Autodesk Fusion 360 part; units mm, degrees
note: some values were not read from the file. Set by a fixed rule: which sketch regions a step uses.
(part 37 of 59)
  spline S18 degree 5 poles (-22.1904, -6.2406) (-22.1905, -6.2407) (-22.1907, -6.2408) (-22.1909, -6.241) (-22.1913, -6.2414) (-22.1919, -6.2419) (-22.1925, -6.2424) (-22.1933, -6.2431) (-22.1941, -6.2438) (-22.195, -6.2446) (-22.196, -6.2455) (-22.197, -6.2464) (-22.1982, -6.2474) (-22.1994, -6.2485) (-22.2007, -6.2497) (-22.202, -6.2509) (-22.2035, -6.2522) (-22.205, -6.2536) (-22.2066, -6.255) (-22.2082, -6.2565) (-22.2099, -6.2581) (-22.2117, -6.2597) (-22.2136, -6.2615) (-22.2155, -6.2632) (-22.2175, -6.2651) (-22.2195, -6.267) (-22.2216, -6.269) (-22.2238, -6.271) (-22.226, -6.2732) (-22.2283, -6.2753) (-22.2307, -6.2776) (-22.2331, -6.2799) (-22.2355, -6.2823) (-22.238, -6.2847) (-22.2406, -6.2872) (-22.2433, -6.2897) (-22.2459, -6.2924) (-22.2487, -6.2951) (-22.2515, -6.2978) (-22.2543, -6.3006) (-22.2572, -6.3035) (-22.2602, -6.3064) (-22.2632, -6.3094) (-22.2662, -6.3124) (-22.2693, -6.3156) (-22.2725, -6.3187) (-22.2757, -6.322) (-22.2789, -6.3252) (-22.2822, -6.3286) (-22.2855, -6.332) (-22.2889, -6.3355) (-22.2923, -6.339) (-22.2958, -6.3426) (-22.2993, -6.3462) (-22.3029, -6.3499) (-22.3065, -6.3536) (-22.3101, -6.3574) (-22.3138, -6.3613) (-22.3175, -6.3652) (-22.3212, -6.3692) (-22.325, -6.3732) (-22.3289, -6.3773) (-22.3328, -6.3814) (-22.3367, -6.3856) (-22.3406, -6.3899) (-22.3446, -6.3942) (-22.3486, -6.3986) (-22.3527, -6.403) (-22.3568, -6.4074) (-22.3609, -6.4119) (-22.3651, -6.4165) (-22.3693, -6.4211) (-22.3736, -6.4258) (-22.3778, -6.4306) (-22.3821, -6.4353) (-22.3865, -6.4402) (-22.3909, -6.4451) (-22.3953, -6.45) (-22.3997, -6.455) (-22.4042, -6.46) (-22.4087, -6.4651) (-22.4132, -6.4703) (-22.4177, -6.4755) (-22.4223, -6.4807) (-22.427, -6.486) (-22.4316, -6.4914) (-22.4363, -6.4968) (-22.441, -6.5022) (-22.4457, -6.5077) (-22.4505, -6.5133) (-22.4553, -6.5189) (-22.4601, -6.5246) (-22.4649, -6.5303) (-22.4698, -6.536) (-22.4747, -6.5418) (-22.4796, -6.5477) (-22.4846, -6.5536) (-22.4895, -6.5595) (-22.4945, -6.5655) (-22.4996, -6.5715) (-22.5046, -6.5776) (-22.5097, -6.5838) (-22.5148, -6.59) (-22.5199, -6.5962) (-22.525, -6.6025) (-22.5302, -6.6088) (-22.5354, -6.6152) (-22.5406, -6.6216) (-22.5458, -6.6281) (-22.5511, -6.6346) (-22.5564, -6.6412) (-22.5617, -6.6478) (-22.567, -6.6544) (-22.5723, -6.6611) (-22.5777, -6.6679) (-22.583, -6.6747) (-22.5884, -6.6815) (-22.5939, -6.6884) (-22.5993, -6.6954) (-22.6048, -6.7024) (-22.6102, -6.7094) (-22.6157, -6.7165) (-22.6212, -6.7236) (-22.6268, -6.7307) (-22.6323, -6.7379) (-22.6379, -6.7452) (-22.6435, -6.7525) (-22.6491, -6.7598) (-22.6547, -6.7672) (-22.6603, -6.7747) (-22.666, -6.7821) (-22.6716, -6.7897) (-22.6773, -6.7972) (-22.683, -6.8048) (-22.6887, -6.8125) (-22.6945, -6.8202) (-22.7002, -6.8279) (-22.706, -6.8357) (-22.7118, -6.8436) (-22.7175, -6.8514) (-22.7233, -6.8593) (-22.7292, -6.8673) (-22.735, -6.8753) (-22.7408, -6.8834) (-22.7467, -6.8914) (-22.7526, -6.8996) (-22.7585, -6.9078) (-22.7644, -6.916) (-22.7703, -6.9242) (-22.7762, -6.9325) (-22.7822, -6.9409) (-22.7881, -6.9493) (-22.7941, -6.9577) (-22.8, -6.9662) (-22.806, -6.9747) (-22.812, -6.9832) (-22.818, -6.9918) (-22.8241, -7.0005) (-22.8301, -7.0091) (-22.8361, -7.0179) (-22.8422, -7.0266) (-22.8483, -7.0354) (-22.8543, -7.0443) (-22.8604, -7.0532) (-22.8665, -7.0621) (-22.8726, -7.0711) (-22.8787, -7.0801) (-22.8849, -7.0891) (-22.891, -7.0982) (-22.8971, -7.1073) (-22.9033, -7.1165) (-22.9095, -7.1257) (-22.9156, -7.135) (-22.9218, -7.1443) (-22.928, -7.1536) (-22.9342, -7.163) (-22.9404, -7.1724) (-22.9466, -7.1818) (-22.9528, -7.1913) (-22.9591, -7.2009) (-22.9653, -7.2104) (-22.9715, -7.22) (-22.9778, -7.2297) (-22.984, -7.2394) (-22.9903, -7.2491) (-22.9966, -7.2589) (-23.0029, -7.2687) (-23.0091, -7.2785) (-23.0154, -7.2884) (-23.0217, -7.2984) (-23.028, -7.3083) (-23.0343, -7.3183) (-23.0406, -7.3284) (-23.047, -7.3384) (-23.0533, -7.3486) (-23.0596, -7.3587) (-23.066, -7.3689) (-23.0723, -7.3791) (-23.0786, -7.3894) (-23.085, -7.3997) (-23.0914, -7.4101) (-23.0977, -7.4205) (-23.1041, -7.4309) (-23.1104, -7.4413) (-23.1168, -7.4518) (-23.1232, -7.4624) (-23.1296, -7.473) (-23.136, -7.4836) (-23.1423, -7.4942) (-23.1487, -7.5049) (-23.1551, -7.5156) (-23.1615, -7.5264) (-23.1679, -7.5372) (-23.1743, -7.548) (-23.1807, -7.5589) (-23.1872, -7.5698) (-23.1936, -7.5808) (-23.2, -7.5917) (-23.2064, -7.6028) (-23.2128, -7.6138) (-23.2193, -7.6249) (-23.2257, -7.636) (-23.2321, -7.6472) (-23.2385, -7.6584) (-23.245, -7.6697) (-23.2514, -7.6809) (-23.2578, -7.6922) (-23.2643, -7.7036) (-23.2707, -7.715) (-23.2771, -7.7264) (-23.2836, -7.7379) (-23.29, -7.7493) (-23.2965, -7.7609) (-23.3029, -7.7724) (-23.3094, -7.784) (-23.3158, -7.7957) (-23.3222, -7.8073) (-23.3287, -7.819) (-23.3351, -7.8308) (-23.3416, -7.8426) (-23.348, -7.8544) (-23.3532, -7.8639) (-23.3571, -7.871) (-23.3596, -7.8757) (-23.3609, -7.8781) knots 0 0 0 0 0 0 0.00416667 0.00833333 0.0125 0.01666667 0.02083333 0.025 0.02916667 0.03333333 0.0375 0.04166667 0.04583333 0.05 0.05416667 0.05833333 0.0625 0.06666667 0.07083333 0.075 0.07916667 0.08333333 0.0875 0.09166667 0.09583333 0.1 0.10416667 0.10833333 0.1125 0.11666667 0.12083333 0.125 0.12916667 0.13333333 0.1375 0.14166667 0.14583333 0.15 0.15416667 0.15833333 0.1625 0.16666667 0.17083333 0.175 0.17916667 0.18333333 0.1875 0.19166667 0.19583333 0.2 0.20416667 0.20833333 0.2125 0.21666667 0.22083333 0.225 0.22916667 0.23333333 0.2375 0.24166667 0.24583333 0.25 0.25416667 0.25833333 0.2625 0.26666667 0.27083333 0.275 0.27916667 0.28333333 0.2875 0.29166667 0.29583333 0.3 0.30416667 0.30833333 0.3125 0.31666667 0.32083333 0.325 0.32916667 0.33333333 0.3375 0.34166667 0.34583333 0.35 0.35416667 0.35833333 0.3625 0.36666667 0.37083333 0.375 0.37916667 0.38333333 0.3875 0.39166667 0.39583333 0.4 0.40416667 0.40833333 0.4125 0.41666667 0.42083333 0.425 0.42916667 0.43333333 0.4375 0.44166667 0.44583333 0.45 0.45416667 0.45833333 0.4625 0.46666667 0.47083333 0.475 0.47916667 0.48333333 0.4875 0.49166667 0.49583333 0.5 0.50416667 0.50833333 0.5125 0.51666667 0.52083333 0.525 0.52916667 0.53333333 0.5375 0.54166667 0.54583333 0.55 0.55416667 0.55833333 0.5625 0.56666667 0.57083333 0.575 0.57916667 0.58333333 0.5875 0.59166667 0.59583333 0.6 0.60416667 0.60833333 0.6125 0.61666667 0.62083333 0.625 0.62916667 0.63333333 0.6375 0.64166667 0.64583333 0.65 0.65416667 0.65833333 0.6625 0.66666667 0.67083333 0.675 0.67916667 0.68333333 0.6875 0.69166667 0.69583333 0.7 0.70416667 0.70833333 0.7125 0.71666667 0.72083333 0.725 0.72916667 0.73333333 0.7375 0.74166667 0.74583333 0.75 0.75416667 0.75833333 0.7625 0.76666667 0.77083333 0.775 0.77916667 0.78333333 0.7875 0.79166667 0.79583333 0.8 0.80416667 0.80833333 0.8125 0.81666667 0.82083333 0.825 0.82916667 0.83333333 0.8375 0.84166667 0.84583333 0.85 0.85416667 0.85833333 0.8625 0.86666667 0.87083333 0.875 0.87916667 0.88333333 0.8875 0.89166667 0.89583333 0.9 0.90416667 0.90833333 0.9125 0.91666667 0.92083333 0.925 0.92916667 0.93333333 0.9375 0.94166667 0.94583333 0.95 0.95416667 0.95833333 0.9625 0.96666667 0.97083333 0.975 0.97916667 0.98333333 0.9875 0.99166667 0.99583333 1 1 1 1 1 1
  arc A19 (-23.3609, -7.8781) -> (-22.7084, -8.6029) centre (0, 12.5) ccw
  spline S19 degree 5 poles (-22.7084, -8.6029) (-22.7059, -8.6018) (-22.7009, -8.5998) (-22.6934, -8.5967) (-22.6834, -8.5925) (-22.671, -8.5873) (-22.6586, -8.5822) (-22.6462, -8.577) (-22.6339, -8.5718) (-22.6217, -8.5666) (-22.6094, -8.5614) (-22.5972, -8.5562) (-22.585, -8.551) (-22.5729, -8.5458) (-22.5608, -8.5406) (-22.5487, -8.5354) (-22.5367, -8.5302) (-22.5247, -8.525) (-22.5127, -8.5198) (-22.5008, -8.5145) (-22.4889, -8.5093) (-22.4771, -8.5041) (-22.4653, -8.4989) (-22.4535, -8.4937) (-22.4417, -8.4884) (-22.43, -8.4832) (-22.4184, -8.478) (-22.4067, -8.4727) (-22.3951, -8.4675) (-22.3836, -8.4623) (-22.3721, -8.457) (-22.3606, -8.4518) (-22.3491, -8.4466) (-22.3377, -8.4413) (-22.3264, -8.4361) (-22.315, -8.4308) (-22.3037, -8.4256) (-22.2925, -8.4204) (-22.2812, -8.4151) (-22.2701, -8.4099) (-22.2589, -8.4046) (-22.2478, -8.3994) (-22.2367, -8.3942) (-22.2257, -8.3889) (-22.2147, -8.3837) (-22.2038, -8.3784) (-22.1928, -8.3732) (-22.182, -8.368) (-22.1711, -8.3627) (-22.1603, -8.3575) (-22.1496, -8.3523) (-22.1388, -8.347) (-22.1281, -8.3418) (-22.1175, -8.3366) (-22.1069, -8.3313) (-22.0963, -8.3261) (-22.0858, -8.3209) (-22.0753, -8.3157) (-22.0649, -8.3105) (-22.0544, -8.3052) (-22.0441, -8.3) (-22.0337, -8.2948) (-22.0235, -8.2896) (-22.0132, -8.2844) (-22.003, -8.2792) (-21.9928, -8.274) (-21.9827, -8.2688) (-21.9726, -8.2636) (-21.9625, -8.2584) (-21.9525, -8.2532) (-21.9426, -8.248) (-21.9326, -8.2429) (-21.9228, -8.2377) (-21.9129, -8.2325) (-21.9031, -8.2274) (-21.8933, -8.2222) (-21.8836, -8.217) (-21.8739, -8.2119) (-21.8643, -8.2067) (-21.8547, -8.2016) (-21.8451, -8.1965) (-21.8356, -8.1913) (-21.8261, -8.1862) (-21.8167, -8.1811) (-21.8073, -8.176) (-21.798, -8.1709) (-21.7887, -8.1658) (-21.7794, -8.1607) (-21.7702, -8.1556) (-21.761, -8.1505) (-21.7519, -8.1454) (-21.7428, -8.1404) (-21.7337, -8.1353) (-21.7247, -8.1303) (-21.7158, -8.1252) (-21.7068, -8.1202) (-21.698, -8.1152) (-21.6891, -8.1101) (-21.6803, -8.1051) (-21.6716, -8.1001) (-21.6629, -8.0951) (-21.6542, -8.0902) (-21.6456, -8.0852) (-21.6371, -8.0802) (-21.6285, -8.0753) (-21.6201, -8.0703) (-21.6116, -8.0654) (-21.6032, -8.0605) (-21.5949, -8.0555) (-21.5866, -8.0506) (-21.5783, -8.0457) (-21.5701, -8.0409) (-21.5619, -8.036) (-21.5538, -8.0311) (-21.5458, -8.0263) (-21.5377, -8.0214) (-21.5297, -8.0166) (-21.5218, -8.0118) (-21.5139, -8.007) (-21.5061, -8.0022) (-21.4983, -7.9974) (-21.4905, -7.9927) (-21.4828, -7.9879) (-21.4752, -7.9832) (-21.4676, -7.9784) (-21.46, -7.9737) (-21.4525, -7.969) (-21.445, -7.9644) (-21.4376, -7.9597) (-21.4302, -7.955) (-21.4229, -7.9504) (-21.4156, -7.9458) (-21.4084, -7.9412) (-21.4012, -7.9366) (-21.3941, -7.932) (-21.387, -7.9274) (-21.38, -7.9229) (-21.373, -7.9184) (-21.3661, -7.9139) (-21.3592, -7.9094) (-21.3523, -7.9049) (-21.3455, -7.9004) (-21.3388, -7.896) (-21.3321, -7.8916) (-21.3255, -7.8872) (-21.3189, -7.8828) (-21.3124, -7.8784) (-21.3059, -7.8741) (-21.2995, -7.8698) (-21.2931, -7.8655) (-21.2867, -7.8612) (-21.2805, -7.8569) (-21.2742, -7.8527) (-21.2681, -7.8484) (-21.2619, -7.8442) (-21.2559, -7.8401) (-21.2498, -7.8359) (-21.2439, -7.8318) (-21.238, -7.8277) (-21.2321, -7.8236) (-21.2263, -7.8195) (-21.2205, -7.8155) (-21.2148, -7.8115) (-21.2092, -7.8075) (-21.2036, -7.8035) (-21.1981, -7.7996) (-21.1926, -7.7956) (-21.1871, -7.7918) (-21.1818, -7.7879) (-21.1764, -7.7841) (-21.1712, -7.7802) (-21.166, -7.7765) (-21.1608, -7.7727) (-21.1557, -7.769) (-21.1507, -7.7653) (-21.1457, -7.7616) (-21.1408, -7.758) (-21.1359, -7.7544) (-21.1311, -7.7508) (-21.1263, -7.7472) (-21.1216, -7.7437) (-21.117, -7.7402) (-21.1124, -7.7368) (-21.1079, -7.7333) (-21.1034, -7.73) (-21.099, -7.7266) (-21.0947, -7.7233) (-21.0904, -7.72) (-21.0862, -7.7167) (-21.082, -7.7135) (-21.0779, -7.7103) (-21.0739, -7.7072) (-21.0699, -7.7041) (-21.066, -7.701) (-21.0621, -7.698) (-21.0583, -7.695) (-21.0546, -7.692) (-21.0509, -7.6891) (-21.0473, -7.6862) (-21.0437, -7.6834) (-21.0403, -7.6806) (-21.0368, -7.6778) (-21.0335, -7.6751) (-21.0302, -7.6724) (-21.027, -7.6698) (-21.0238, -7.6672) (-21.0207, -7.6647) (-21.0177, -7.6622) (-21.0148, -7.6597) (-21.0119, -7.6573) (-21.009, -7.655) (-21.0063, -7.6527) (-21.0036, -7.6504) (-21.001, -7.6482) (-20.9984, -7.6461) (-20.996, -7.644) (-20.9936, -7.6419) (-20.9912, -7.6399) (-20.989, -7.638) (-20.9868, -7.6361) (-20.9847, -7.6343) (-20.9826, -7.6325) (-20.9806, -7.6308) (-20.9787, -7.6291) (-20.9769, -7.6275) (-20.9752, -7.626) (-20.9735, -7.6245) (-20.9719, -7.623) (-20.9704, -7.6217) (-20.9689, -7.6204) (-20.9675, -7.6192) (-20.9663, -7.618) (-20.9651, -7.6169) (-20.9639, -7.6159) (-20.9629, -7.6149) (-20.9619, -7.614) (-20.961, -7.6132) (-20.9602, -7.6125) (-20.9595, -7.6118) (-20.9589, -7.6112) (-20.9583, -7.6107) (-20.958, -7.6104) (-20.9577, -7.6102) (-20.9576, -7.61) (-20.9575, -7.61) knots -1 -1 -1 -1 -1 -1 -0.99583333 -0.99166667 -0.9875 -0.98333333 -0.97916667 -0.975 -0.97083333 -0.96666667 -0.9625 -0.95833333 -0.95416667 -0.95 -0.94583333 -0.94166667 -0.9375 -0.93333333 -0.92916667 -0.925 -0.92083333 -0.91666667 -0.9125 -0.90833333 -0.90416667 -0.9 -0.89583333 -0.89166667 -0.8875 -0.88333333 -0.87916667 -0.875 -0.87083333 -0.86666667 -0.8625 -0.85833333 -0.85416667 -0.85 -0.84583333 -0.84166667 -0.8375 -0.83333333 -0.82916667 -0.825 -0.82083333 -0.81666667 -0.8125 -0.80833333 -0.80416667 -0.8 -0.79583333 -0.79166667 -0.7875 -0.78333333 -0.77916667 -0.775 -0.77083333 -0.76666667 -0.7625 -0.75833333 -0.75416667 -0.75 -0.74583333 -0.74166667 -0.7375 -0.73333333 -0.72916667 -0.725 -0.72083333 -0.71666667 -0.7125 -0.70833333 -0.70416667 -0.7 -0.69583333 -0.69166667 -0.6875 -0.68333333 -0.67916667 -0.675 -0.67083333 -0.66666667 -0.6625 -0.65833333 -0.65416667 -0.65 -0.64583333 -0.64166667 -0.6375 -0.63333333 -0.62916667 -0.625 -0.62083333 -0.61666667 -0.6125 -0.60833333 -0.60416667 -0.6 -0.59583333 -0.59166667 -0.5875 -0.58333333 -0.57916667 -0.575 -0.57083333 -0.56666667 -0.5625 -0.55833333 -0.55416667 -0.55 -0.54583333 -0.54166667 -0.5375 -0.53333333 -0.52916667 -0.525 -0.52083333 -0.51666667 -0.5125 -0.50833333 -0.50416667 -0.5 -0.49583333 -0.49166667 -0.4875 -0.48333333 -0.47916667 -0.475 -0.47083333 -0.46666667 -0.4625 -0.45833333 -0.45416667 -0.45 -0.44583333 -0.44166667 -0.4375 -0.43333333 -0.42916667 -0.425 -0.42083333 -0.41666667 -0.4125 -0.40833333 -0.40416667 -0.4 -0.39583333 -0.39166667 -0.3875 -0.38333333 -0.37916667 -0.375 -0.37083333 -0.36666667 -0.3625 -0.35833333 -0.35416667 -0.35 -0.34583333 -0.34166667 -0.3375 -0.33333333 -0.32916667 -0.325 -0.32083333 -0.31666667 -0.3125 -0.30833333 -0.30416667 -0.3 -0.29583333 -0.29166667 -0.2875 -0.28333333 -0.27916667 -0.275 -0.27083333 -0.26666667 -0.2625 -0.25833333 -0.25416667 -0.25 -0.24583333 -0.24166667 -0.2375 -0.23333333 -0.22916667 -0.225 -0.22083333 -0.21666667 -0.2125 -0.20833333 -0.20416667 -0.2 -0.19583333 -0.19166667 -0.1875 -0.18333333 -0.17916667 -0.175 -0.17083333 -0.16666667 -0.1625 -0.15833333 -0.15416667 -0.15 -0.14583333 -0.14166667 -0.1375 -0.13333333 -0.12916667 -0.125 -0.12083333 -0.11666667 -0.1125 -0.10833333 -0.10416667 -0.1 -0.09583333 -0.09166667 -0.0875 -0.08333333 -0.07916667 -0.075 -0.07083333 -0.06666667 -0.0625 -0.05833333 -0.05416667 -0.05 -0.04583333 -0.04166667 -0.0375 -0.03333333 -0.02916667 -0.025 -0.02083333 -0.01666667 -0.0125 -0.00833333 -0.00416667 0 0 0 0 0 0
  line L47 (-20.9575, -7.61) -> (-20.9569, -7.6094)
  line L48 (-20.9569, -7.6094) -> (-20.7445, -7.4055)
  arc A20 (-20.7445, -7.4055) -> (-19.9055, -8.2445) centre (0, 12.5) ccw
  line L49 (-19.9055, -8.2445) -> (-20.1094, -8.4569)
  line L50 (-20.1094, -8.4569) -> (-20.11, -8.4575)
  spline S20 degree 5 poles (-20.11, -8.4575) (-20.11, -8.4576) (-20.1102, -8.4577) (-20.1104, -8.458) (-20.1107, -8.4583) (-20.1112, -8.4589) (-20.1118, -8.4595) (-20.1125, -8.4602) (-20.1132, -8.461) (-20.114, -8.4619) (-20.1149, -8.4629) (-20.1159, -8.4639) (-20.1169, -8.4651) (-20.118, -8.4663) (-20.1192, -8.4675) (-20.1204, -8.4689) (-20.1217, -8.4704) (-20.123, -8.4719) (-20.1245, -8.4735) (-20.126, -8.4752) (-20.1275, -8.4769) (-20.1291, -8.4787) (-20.1308, -8.4806) (-20.1325, -8.4826) (-20.1343, -8.4847) (-20.1361, -8.4868) (-20.138, -8.489) (-20.1399, -8.4912) (-20.1419, -8.4936) (-20.144, -8.496) (-20.1461, -8.4984) (-20.1482, -8.501) (-20.1504, -8.5036) (-20.1527, -8.5063) (-20.155, -8.509) (-20.1573, -8.5119) (-20.1597, -8.5148) (-20.1622, -8.5177) (-20.1647, -8.5207) (-20.1672, -8.5238) (-20.1698, -8.527) (-20.1724, -8.5302) (-20.1751, -8.5335) (-20.1778, -8.5368) (-20.1806, -8.5403) (-20.1834, -8.5437) (-20.1862, -8.5473) (-20.1891, -8.5509) (-20.192, -8.5546) (-20.195, -8.5583) (-20.198, -8.5621) (-20.201, -8.566) (-20.2041, -8.5699) (-20.2072, -8.5739) (-20.2103, -8.5779) (-20.2135, -8.582) (-20.2167, -8.5862) (-20.22, -8.5904) (-20.2233, -8.5947) (-20.2266, -8.599) (-20.23, -8.6034) (-20.2333, -8.6079) (-20.2368, -8.6124) (-20.2402, -8.617) (-20.2437, -8.6216) (-20.2472, -8.6263) (-20.2508, -8.6311) (-20.2544, -8.6359) (-20.258, -8.6408) (-20.2616, -8.6457) (-20.2653, -8.6507) (-20.269, -8.6557) (-20.2727, -8.6608) (-20.2765, -8.666) (-20.2802, -8.6712) (-20.2841, -8.6764) (-20.2879, -8.6818) (-20.2918, -8.6871) (-20.2956, -8.6926) (-20.2996, -8.6981) (-20.3035, -8.7036) (-20.3075, -8.7092) (-20.3115, -8.7148) (-20.3155, -8.7205) (-20.3195, -8.7263) (-20.3236, -8.7321) (-20.3277, -8.738) (-20.3318, -8.7439) (-20.3359, -8.7498) (-20.3401, -8.7559) (-20.3442, -8.7619) (-20.3484, -8.7681) (-20.3527, -8.7742) (-20.3569, -8.7805) (-20.3612, -8.7867) (-20.3655, -8.7931) (-20.3698, -8.7995) (-20.3741, -8.8059) (-20.3784, -8.8124) (-20.3828, -8.8189) (-20.3872, -8.8255) (-20.3916, -8.8321) (-20.396, -8.8388) (-20.4004, -8.8455) (-20.4049, -8.8523) (-20.4094, -8.8592) (-20.4139, -8.8661) (-20.4184, -8.873) (-20.4229, -8.88) (-20.4274, -8.887) (-20.432, -8.8941) (-20.4366, -8.9012) (-20.4412, -8.9084) (-20.4458, -8.9156) (-20.4504, -8.9229) (-20.455, -8.9302) (-20.4597, -8.9376) (-20.4644, -8.945) (-20.469, -8.9525) (-20.4737, -8.96) (-20.4784, -8.9676) (-20.4832, -8.9752) (-20.4879, -8.9828) (-20.4927, -8.9905) (-20.4974, -8.9983) (-20.5022, -9.0061) (-20.507, -9.0139) (-20.5118, -9.0218) (-20.5166, -9.0297) (-20.5214, -9.0377) (-20.5263, -9.0458) (-20.5311, -9.0538) (-20.536, -9.0619) (-20.5409, -9.0701) (-20.5457, -9.0783) (-20.5506, -9.0866) (-20.5555, -9.0949) (-20.5605, -9.1032) (-20.5654, -9.1116) (-20.5703, -9.1201) (-20.5753, -9.1285) (-20.5802, -9.1371) (-20.5852, -9.1456) (-20.5902, -9.1542) (-20.5951, -9.1629) (-20.6001, -9.1716) (-20.6051, -9.1803) (-20.6101, -9.1891) (-20.6152, -9.198) (-20.6202, -9.2068) (-20.6252, -9.2158) (-20.6303, -9.2247) (-20.6353, -9.2337) (-20.6404, -9.2428) (-20.6454, -9.2519) (-20.6505, -9.261) (-20.6556, -9.2702) (-20.6607, -9.2794) (-20.6658, -9.2887) (-20.6709, -9.298) (-20.676, -9.3073) (-20.6811, -9.3167) (-20.6862, -9.3261) (-20.6913, -9.3356) (-20.6965, -9.3451) (-20.7016, -9.3547) (-20.7067, -9.3643) (-20.7119, -9.3739) (-20.717, -9.3836) (-20.7222, -9.3933) (-20.7274, -9.4031) (-20.7325, -9.4129) (-20.7377, -9.4228) (-20.7429, -9.4326) (-20.748, -9.4426) (-20.7532, -9.4525) (-20.7584, -9.4625) (-20.7636, -9.4726) (-20.7688, -9.4827) (-20.774, -9.4928) (-20.7792, -9.503) (-20.7844, -9.5132) (-20.7896, -9.5235) (-20.7948, -9.5337) (-20.8, -9.5441) (-20.8052, -9.5544) (-20.8105, -9.5649) (-20.8157, -9.5753) (-20.8209, -9.5858) (-20.8261, -9.5963) (-20.8313, -9.6069) (-20.8366, -9.6175) (-20.8418, -9.6281) (-20.847, -9.6388) (-20.8523, -9.6496) (-20.8575, -9.6603) (-20.8627, -9.6711) (-20.868, -9.682) (-20.8732, -9.6928) (-20.8784, -9.7038) (-20.8837, -9.7147) (-20.8889, -9.7257) (-20.8942, -9.7367) (-20.8994, -9.7478) (-20.9046, -9.7589) (-20.9099, -9.7701) (-20.9151, -9.7812) (-20.9204, -9.7925) (-20.9256, -9.8037) (-20.9308, -9.815) (-20.9361, -9.8264) (-20.9413, -9.8377) (-20.9466, -9.8491) (-20.9518, -9.8606) (-20.957, -9.8721) (-20.9623, -9.8836) (-20.9675, -9.8951) (-20.9727, -9.9067) (-20.978, -9.9184) (-20.9832, -9.93) (-20.9884, -9.9417) (-20.9937, -9.9535) (-20.9989, -9.9653) (-21.0041, -9.9771) (-21.0093, -9.9889) (-21.0145, -10.0008) (-21.0198, -10.0127) (-21.025, -10.0247) (-21.0302, -10.0367) (-21.0354, -10.0487) (-21.0406, -10.0608) (-21.0458, -10.0729) (-21.051, -10.085) (-21.0562, -10.0972) (-21.0614, -10.1094) (-21.0666, -10.1217) (-21.0718, -10.1339) (-21.077, -10.1462) (-21.0822, -10.1586) (-21.0873, -10.171) (-21.0925, -10.1834) (-21.0967, -10.1934) (-21.0998, -10.2009) (-21.1018, -10.2059) (-21.1029, -10.2084) knots 0 0 0 0 0 0 0.00416667 0.00833333 0.0125 0.01666667 0.02083333 0.025 0.02916667 0.03333333 0.0375 0.04166667 0.04583333 0.05 0.05416667 0.05833333 0.0625 0.06666667 0.07083333 0.075 0.07916667 0.08333333 0.0875 0.09166667 0.09583333 0.1 0.10416667 0.10833333 0.1125 0.11666667 0.12083333 0.125 0.12916667 0.13333333 0.1375 0.14166667 0.14583333 0.15 0.15416667 0.15833333 0.1625 0.16666667 0.17083333 0.175 0.17916667 0.18333333 0.1875 0.19166667 0.19583333 0.2 0.20416667 0.20833333 0.2125 0.21666667 0.22083333 0.225 0.22916667 0.23333333 0.2375 0.24166667 0.24583333 0.25 0.25416667 0.25833333 0.2625 0.26666667 0.27083333 0.275 0.27916667 0.28333333 0.2875 0.29166667 0.29583333 0.3 0.30416667 0.30833333 0.3125 0.31666667 0.32083333 0.325 0.32916667 0.33333333 0.3375 0.34166667 0.34583333 0.35 0.35416667 0.35833333 0.3625 0.36666667 0.37083333 0.375 0.37916667 0.38333333 0.3875 0.39166667 0.39583333 0.4 0.40416667 0.40833333 0.4125 0.41666667 0.42083333 0.425 0.42916667 0.43333333 0.4375 0.44166667 0.44583333 0.45 0.45416667 0.45833333 0.4625 0.46666667 0.47083333 0.475 0.47916667 0.48333333 0.4875 0.49166667 0.49583333 0.5 0.50416667 0.50833333 0.5125 0.51666667 0.52083333 0.525 0.52916667 0.53333333 0.5375 0.54166667 0.54583333 0.55 0.55416667 0.55833333 0.5625 0.56666667 0.57083333 0.575 0.57916667 0.58333333 0.5875 0.59166667 0.59583333 0.6 0.60416667 0.60833333 0.6125 0.61666667 0.62083333 0.625 0.62916667 0.63333333 0.6375 0.64166667 0.64583333 0.65 0.65416667 0.65833333 0.6625 0.66666667 0.67083333 0.675 0.67916667 0.68333333 0.6875 0.69166667 0.69583333 0.7 0.70416667 0.70833333 0.7125 0.71666667 0.72083333 0.725 0.72916667 0.73333333 0.7375 0.74166667 0.74583333 0.75 0.75416667 0.75833333 0.7625 0.76666667 0.77083333 0.775 0.77916667 0.78333333 0.7875 0.79166667 0.79583333 0.8 0.80416667 0.80833333 0.8125 0.81666667 0.82083333 0.825 0.82916667 0.83333333 0.8375 0.84166667 0.84583333 0.85 0.85416667 0.85833333 0.8625 0.86666667 0.87083333 0.875 0.87916667 0.88333333 0.8875 0.89166667 0.89583333 0.9 0.90416667 0.90833333 0.9125 0.91666667 0.92083333 0.925 0.92916667 0.93333333 0.9375 0.94166667 0.94583333 0.95 0.95416667 0.95833333 0.9625 0.96666667 0.97083333 0.975 0.97916667 0.98333333 0.9875 0.99166667 0.99583333 1 1 1 1 1 1
  arc A21 (-21.1029, -10.2084) -> (-20.3781, -10.8609) centre (0, 12.5) ccw
  spline S21 degree 5 poles (-20.3781, -10.8609) (-20.3757, -10.8596) (-20.371, -10.8571) (-20.3639, -10.8532) (-20.3544, -10.848) (-20.3426, -10.8416) (-20.3308, -10.8351) (-20.319, -10.8287) (-20.3073, -10.8222) (-20.2957, -10.8158) (-20.284, -10.8094) (-20.2724, -10.8029) (-20.2609, -10.7965) (-20.2493, -10.79) (-20.2379, -10.7836) (-20.2264, -10.7771) (-20.215, -10.7707) (-20.2036, -10.7643) (-20.1922, -10.7578) (-20.1809, -10.7514) (-20.1697, -10.745) (-20.1584, -10.7385) (-20.1472, -10.7321) (-20.136, -10.7257) (-20.1249, -10.7193) (-20.1138, -10.7128) (-20.1028, -10.7064) (-20.0917, -10.7) (-20.0808, -10.6936) (-20.0698, -10.6872) (-20.0589, -10.6807) (-20.048, -10.6743) (-20.0372, -10.6679) (-20.0264, -10.6615) (-20.0156, -10.6551) (-20.0049, -10.6487) (-19.9942, -10.6423) (-19.9836, -10.636) (-19.973, -10.6296) (-19.9624, -10.6232) (-19.9518, -10.6168) (-19.9413, -10.6104) (-19.9309, -10.6041) (-19.9205, -10.5977) (-19.9101, -10.5914) (-19.8997, -10.585) (-19.8894, -10.5786) (-19.8791, -10.5723) (-19.8689, -10.566) (-19.8587, -10.5596) (-19.8486, -10.5533) (-19.8384, -10.547) (-19.8284, -10.5406) (-19.8183, -10.5343) (-19.8083, -10.528) (-19.7984, -10.5217) (-19.7884, -10.5154) (-19.7785, -10.5091) (-19.7687, -10.5029) (-19.7589, -10.4966) (-19.7491, -10.4903) (-19.7394, -10.484) (-19.7297, -10.4778) (-19.72, -10.4715) (-19.7104, -10.4653) (-19.7009, -10.4591) (-19.6913, -10.4528) (-19.6818, -10.4466) (-19.6724, -10.4404) (-19.663, -10.4342) (-19.6536, -10.428) (-19.6443, -10.4218) (-19.635, -10.4156) (-19.6257, -10.4095) (-19.6165, -10.4033) (-19.6073, -10.3971) (-19.5982, -10.391) (-19.5891, -10.3849) (-19.5801, -10.3787) (-19.5711, -10.3726) (-19.5621, -10.3665) (-19.5532, -10.3604) (-19.5443, -10.3543) (-19.5354, -10.3483) (-19.5266, -10.3422) (-19.5179, -10.3361) (-19.5091, -10.3301) (-19.5005, -10.3241) (-19.4918, -10.318) (-19.4832, -10.312) (-19.4747, -10.306) (-19.4662, -10.3) (-19.4577, -10.2941) (-19.4493, -10.2881) (-19.4409, -10.2822) (-19.4325, -10.2762) (-19.4242, -10.2703) (-19.416, -10.2644) (-19.4078, -10.2585) (-19.3996, -10.2526) (-19.3914, -10.2467) (-19.3834, -10.2408) (-19.3753, -10.235) (-19.3673, -10.2292) (-19.3593, -10.2233) (-19.3514, -10.2175) (-19.3436, -10.2118) (-19.3357, -10.206) (-19.3279, -10.2002) (-19.3202, -10.1945) (-19.3125, -10.1887) (-19.3048, -10.183) (-19.2972, -10.1773) (-19.2897, -10.1716) (-19.2821, -10.166) (-19.2747, -10.1603) (-19.2672, -10.1547) (-19.2598, -10.1491) (-19.2525, -10.1435) (-19.2452, -10.1379) (-19.2379, -10.1323) (-19.2307, -10.1268) (-19.2236, -10.1212) (-19.2165, -10.1157) (-19.2094, -10.1102) (-19.2024, -10.1048) (-19.1954, -10.0993) (-19.1884, -10.0939) (-19.1815, -10.0884) (-19.1747, -10.083) (-19.1679, -10.0777) (-19.1611, -10.0723) (-19.1544, -10.067) (-19.1478, -10.0617) (-19.1412, -10.0564) (-19.1346, -10.0511) (-19.1281, -10.0458) (-19.1216, -10.0406) (-19.1152, -10.0354) (-19.1088, -10.0302) (-19.1025, -10.025) (-19.0962, -10.0199) (-19.09, -10.0148) (-19.0838, -10.0097) (-19.0776, -10.0046) (-19.0715, -9.9996) (-19.0655, -9.9945) (-19.0595, -9.9895) (-19.0536, -9.9846) (-19.0477, -9.9796) (-19.0418, -9.9747) (-19.036, -9.9698) (-19.0303, -9.9649) (-19.0246, -9.9601) (-19.0189, -9.9553) (-19.0133, -9.9505) (-19.0077, -9.9457) (-19.0022, -9.941) (-18.9968, -9.9363) (-18.9914, -9.9316) (-18.986, -9.927) (-18.9807, -9.9223) (-18.9755, -9.9177) (-18.9703, -9.9132) (-18.9651, -9.9087) (-18.96, -9.9042) (-18.955, -9.8997) (-18.95, -9.8953) (-18.9451, -9.8909) (-18.9402, -9.8865) (-18.9353, -9.8821) (-18.9306, -9.8778) (-18.9258, -9.8736) (-18.9211, -9.8693) (-18.9165, -9.8651) (-18.9119, -9.8609) (-18.9074, -9.8568) (-18.903, -9.8527) (-18.8986, -9.8486) (-18.8942, -9.8446) (-18.8899, -9.8406) (-18.8856, -9.8367) (-18.8814, -9.8328) (-18.8773, -9.8289) (-18.8732, -9.825) (-18.8692, -9.8212) (-18.8652, -9.8175) (-18.8613, -9.8138) (-18.8574, -9.8101) (-18.8536, -9.8065) (-18.8499, -9.8029) (-18.8462, -9.7993) (-18.8426, -9.7958) (-18.839, -9.7923) (-18.8355, -9.7889) (-18.832, -9.7855) (-18.8286, -9.7822) (-18.8252, -9.7789) (-18.822, -9.7757) (-18.8187, -9.7725) (-18.8156, -9.7693) (-18.8124, -9.7662) (-18.8094, -9.7632) (-18.8064, -9.7602) (-18.8035, -9.7572) (-18.8006, -9.7543) (-18.7978, -9.7515) (-18.7951, -9.7487) (-18.7924, -9.7459) (-18.7897, -9.7433) (-18.7872, -9.7406) (-18.7847, -9.738) (-18.7823, -9.7355) (-18.7799, -9.7331) (-18.7776, -9.7307) (-18.7753, -9.7283) (-18.7732, -9.726) (-18.771, -9.7238) (-18.769, -9.7216) (-18.767, -9.7195) (-18.7651, -9.7175) (-18.7632, -9.7155) (-18.7615, -9.7136) (-18.7597, -9.7117) (-18.7581, -9.7099) (-18.7565, -9.7082) (-18.755, -9.7066) (-18.7536, -9.705) (-18.7522, -9.7035) (-18.7509, -9.702) (-18.7497, -9.7007) (-18.7485, -9.6994) (-18.7474, -9.6982) (-18.7464, -9.697) (-18.7455, -9.696) (-18.7446, -9.695) (-18.7438, -9.6941) (-18.7431, -9.6933) (-18.7424, -9.6925) (-18.7419, -9.6919) (-18.7414, -9.6913) (-18.741, -9.6909) (-18.7408, -9.6907) (-18.7407, -9.6905) (-18.7406, -9.6904) knots -1 -1 -1 -1 -1 -1 -0.99583333 -0.99166667 -0.9875 -0.98333333 -0.97916667 -0.975 -0.97083333 -0.96666667 -0.9625 -0.95833333 -0.95416667 -0.95 -0.94583333 -0.94166667 -0.9375 -0.93333333 -0.92916667 -0.925 -0.92083333 -0.91666667 -0.9125 -0.90833333 -0.90416667 -0.9 -0.89583333 -0.89166667 -0.8875 -0.88333333 -0.87916667 -0.875 -0.87083333 -0.86666667 -0.8625 -0.85833333 -0.85416667 -0.85 -0.84583333 -0.84166667 -0.8375 -0.83333333 -0.82916667 -0.825 -0.82083333 -0.81666667 -0.8125 -0.80833333 -0.80416667 -0.8 -0.79583333 -0.79166667 -0.7875 -0.78333333 -0.77916667 -0.775 -0.77083333 -0.76666667 -0.7625 -0.75833333 -0.75416667 -0.75 -0.74583333 -0.74166667 -0.7375 -0.73333333 -0.72916667 -0.725 -0.72083333 -0.71666667 -0.7125 -0.70833333 -0.70416667 -0.7 -0.69583333 -0.69166667 -0.6875 -0.68333333 -0.67916667 -0.675 -0.67083333 -0.66666667 -0.6625 -0.65833333 -0.65416667 -0.65 -0.64583333 -0.64166667 -0.6375 -0.63333333 -0.62916667 -0.625 -0.62083333 -0.61666667 -0.6125 -0.60833333 -0.60416667 -0.6 -0.59583333 -0.59166667 -0.5875 -0.58333333 -0.57916667 -0.575 -0.57083333 -0.56666667 -0.5625 -0.55833333 -0.55416667 -0.55 -0.54583333 -0.54166667 -0.5375 -0.53333333 -0.52916667 -0.525 -0.52083333 -0.51666667 -0.5125 -0.50833333 -0.50416667 -0.5 -0.49583333 -0.49166667 -0.4875 -0.48333333 -0.47916667 -0.475 -0.47083333 -0.46666667 -0.4625 -0.45833333 -0.45416667 -0.45 -0.44583333 -0.44166667 -0.4375 -0.43333333 -0.42916667 -0.425 -0.42083333 -0.41666667 -0.4125 -0.40833333 -0.40416667 -0.4 -0.39583333 -0.39166667 -0.3875 -0.38333333 -0.37916667 -0.375 -0.37083333 -0.36666667 -0.3625 -0.35833333 -0.35416667 -0.35 -0.34583333 -0.34166667 -0.3375 -0.33333333 -0.32916667 -0.325 -0.32083333 -0.31666667 -0.3125 -0.30833333 -0.30416667 -0.3 -0.29583333 -0.29166667 -0.2875 -0.28333333 -0.27916667 -0.275 -0.27083333 -0.26666667 -0.2625 -0.25833333 -0.25416667 -0.25 -0.24583333 -0.24166667 -0.2375 -0.23333333 -0.22916667 -0.225 -0.22083333 -0.21666667 -0.2125 -0.20833333 -0.20416667 -0.2 -0.19583333 -0.19166667 -0.1875 -0.18333333 -0.17916667 -0.175 -0.17083333 -0.16666667 -0.1625 -0.15833333 -0.15416667 -0.15 -0.14583333 -0.14166667 -0.1375 -0.13333333 -0.12916667 -0.125 -0.12083333 -0.11666667 -0.1125 -0.10833333 -0.10416667 -0.1 -0.09583333 -0.09166667 -0.0875 -0.08333333 -0.07916667 -0.075 -0.07083333 -0.06666667 -0.0625 -0.05833333 -0.05416667 -0.05 -0.04583333 -0.04166667 -0.0375 -0.03333333 -0.02916667 -0.025 -0.02083333 -0.01666667 -0.0125 -0.00833333 -0.00416667 0 0 0 0 0 0
  line L51 (-18.7406, -9.6904) -> (-18.7401, -9.6898)
  line L52 (-18.7401, -9.6898) -> (-18.5501, -9.4649)
  arc A22 (-18.5501, -9.4649) -> (-17.6281, -10.2115) centre (0, 12.5) ccw
  line L53 (-17.6281, -10.2115) -> (-17.8086, -10.4441)
  line L54 (-17.8086, -10.4441) -> (-17.8091, -10.4448)
  spline S22 degree 5 poles (-17.8091, -10.4448) (-17.8092, -10.4448) (-17.8093, -10.445) (-17.8095, -10.4453) (-17.8098, -10.4457) (-17.8103, -10.4463) (-17.8108, -10.4469) (-17.8114, -10.4477) (-17.812, -10.4486) (-17.8127, -10.4496) (-17.8135, -10.4506) (-17.8144, -10.4518) (-17.8153, -10.453) (-17.8162, -10.4543) (-17.8172, -10.4557) (-17.8183, -10.4572) (-17.8195, -10.4588) (-17.8207, -10.4604) (-17.8219, -10.4622) (-17.8232, -10.464) (-17.8246, -10.4659) (-17.826, -10.4679) (-17.8274, -10.4699) (-17.8289, -10.4721) (-17.8305, -10.4743) (-17.8321, -10.4766) (-17.8337, -10.479) (-17.8354, -10.4814) (-17.8372, -10.484) (-17.8389, -10.4866) (-17.8408, -10.4893) (-17.8427, -10.492) (-17.8446, -10.4948) (-17.8465, -10.4978) (-17.8485, -10.5007) (-17.8506, -10.5038) (-17.8527, -10.5069) (-17.8548, -10.5101) (-17.857, -10.5134) (-17.8592, -10.5167) (-17.8614, -10.5201) (-17.8637, -10.5236) (-17.866, -10.5271) (-17.8683, -10.5308) (-17.8707, -10.5344) (-17.8731, -10.5382) (-17.8756, -10.542) (-17.8781, -10.5459) (-17.8806, -10.5499) (-17.8831, -10.5539) (-17.8857, -10.558) (-17.8883, -10.5621) (-17.891, -10.5664) (-17.8937, -10.5706) (-17.8964, -10.575) (-17.8991, -10.5794) (-17.9019, -10.5839) (-17.9047, -10.5884) (-17.9075, -10.593) (-17.9103, -10.5977) (-17.9132, -10.6024) (-17.9161, -10.6072) (-17.9191, -10.6121) (-17.922, -10.617) (-17.925, -10.622) (-17.928, -10.627) (-17.931, -10.6321) (-17.9341, -10.6373) (-17.9372, -10.6425) (-17.9403, -10.6478) (-17.9434, -10.6531) (-17.9466, -10.6585) (-17.9497, -10.664) (-17.9529, -10.6695) (-17.9562, -10.6751) (-17.9594, -10.6807) (-17.9627, -10.6864) (-17.9659, -10.6921) (-17.9692, -10.6979) (-17.9726, -10.7038) (-17.9759, -10.7097) (-17.9793, -10.7157) (-17.9826, -10.7217) (-17.986, -10.7278) (-17.9895, -10.734) (-17.9929, -10.7402) (-17.9963, -10.7464) (-17.9998, -10.7527) (-18.0033, -10.7591) (-18.0068, -10.7655) (-18.0103, -10.772) (-18.0139, -10.7785) (-18.0174, -10.7851) (-18.021, -10.7918) (-18.0246, -10.7984) (-18.0282, -10.8052) (-18.0318, -10.812) (-18.0354, -10.8188) (-18.039, -10.8257) (-18.0427, -10.8327) (-18.0464, -10.8397) (-18.0501, -10.8468) (-18.0538, -10.8539) (-18.0575, -10.861) (-18.0612, -10.8683) (-18.0649, -10.8755) (-18.0687, -10.8828) (-18.0724, -10.8902) (-18.0762, -10.8976) (-18.08, -10.9051) (-18.0838, -10.9126) (-18.0876, -10.9202) (-18.0914, -10.9278) (-18.0952, -10.9355) (-18.0991, -10.9432) (-18.1029, -10.951) (-18.1068, -10.9588) (-18.1106, -10.9666) (-18.1145, -10.9746) (-18.1184, -10.9825) (-18.1223, -10.9905) (-18.1262, -10.9986) (-18.1301, -11.0067) (-18.134, -11.0149) (-18.1379, -11.0231) (-18.1419, -11.0313) (-18.1458, -11.0396) (-18.1498, -11.048) (-18.1537, -11.0564) (-18.1577, -11.0648) (-18.1617, -11.0733) (-18.1657, -11.0818) (-18.1696, -11.0904) (-18.1736, -11.0991) (-18.1776, -11.1077) (-18.1816, -11.1165) (-18.1857, -11.1252) (-18.1897, -11.134) (-18.1937, -11.1429) (-18.1977, -11.1518) (-18.2018, -11.1607) (-18.2058, -11.1697) (-18.2098, -11.1788) (-18.2139, -11.1879) (-18.2179, -11.197) (-18.222, -11.2062) (-18.226, -11.2154) (-18.2301, -11.2247) (-18.2342, -11.234) (-18.2383, -11.2433) (-18.2423, -11.2527) (-18.2464, -11.2622) (-18.2505, -11.2716) (-18.2546, -11.2812) (-18.2587, -11.2907) (-18.2627, -11.3004) (-18.2668, -11.31) (-18.2709, -11.3197) (-18.275, -11.3295) (-18.2791, -11.3393) (-18.2832, -11.3491) (-18.2873, -11.359) (-18.2914, -11.3689) (-18.2955, -11.3788) (-18.2996, -11.3888) (-18.3038, -11.3989) (-18.3079, -11.409) (-18.312, -11.4191) (-18.3161, -11.4292) (-18.3202, -11.4395) (-18.3243, -11.4497) (-18.3284, -11.46) (-18.3325, -11.4703) (-18.3366, -11.4807) (-18.3408, -11.4911) (-18.3449, -11.5016) (-18.349, -11.5121) (-18.3531, -11.5226) (-18.3572, -11.5332) (-18.3613, -11.5438) (-18.3654, -11.5545) (-18.3695, -11.5652) (-18.3736, -11.5759) (-18.3777, -11.5867) (-18.3818, -11.5975) (-18.3859, -11.6084) (-18.39, -11.6193) (-18.3941, -11.6302) (-18.3982, -11.6412) (-18.4023, -11.6522) (-18.4064, -11.6633) (-18.4105, -11.6744) (-18.4146, -11.6855) (-18.4187, -11.6967) (-18.4228, -11.7079) (-18.4269, -11.7191) (-18.4309, -11.7304) (-18.435, -11.7417) (-18.4391, -11.7531) (-18.4431, -11.7645) (-18.4472, -11.776) (-18.4513, -11.7874) (-18.4553, -11.799) (-18.4594, -11.8105) (-18.4634, -11.8221) (-18.4675, -11.8337) (-18.4715, -11.8454) (-18.4756, -11.8571) (-18.4796, -11.8689) (-18.4836, -11.8806) (-18.4877, -11.8925) (-18.4917, -11.9043) (-18.4957, -11.9162) (-18.4997, -11.9281) (-18.5037, -11.9401) (-18.5077, -11.9521) (-18.5117, -11.9642) (-18.5157, -11.9762) (-18.5197, -11.9884) (-18.5237, -12.0005) (-18.5277, -12.0127) (-18.5316, -12.0249) (-18.5356, -12.0372) (-18.5395, -12.0495) (-18.5435, -12.0618) (-18.5475, -12.0742) (-18.5514, -12.0866) (-18.5553, -12.099) (-18.5593, -12.1115) (-18.5632, -12.124) (-18.5671, -12.1365) (-18.571, -12.1491) (-18.5749, -12.1617) (-18.5788, -12.1744) (-18.5827, -12.1871) (-18.5866, -12.1998) (-18.5905, -12.2125) (-18.5943, -12.2253) (-18.5982, -12.2382) (-18.6021, -12.251) (-18.6059, -12.2639) (-18.609, -12.2743) (-18.6113, -12.282) (-18.6128, -12.2872) (-18.6136, -12.2898) knots 0 0 0 0 0 0 0.00416667 0.00833333 0.0125 0.01666667 0.02083333 0.025 0.02916667 0.03333333 0.0375 0.04166667 0.04583333 0.05 0.05416667 0.05833333 0.0625 0.06666667 0.07083333 0.075 0.07916667 0.08333333 0.0875 0.09166667 0.09583333 0.1 0.10416667 0.10833333 0.1125 0.11666667 0.12083333 0.125 0.12916667 0.13333333 0.1375 0.14166667 0.14583333 0.15 0.15416667 0.15833333 0.1625 0.16666667 0.17083333 0.175 0.17916667 0.18333333 0.1875 0.19166667 0.19583333 0.2 0.20416667 0.20833333 0.2125 0.21666667 0.22083333 0.225 0.22916667 0.23333333 0.2375 0.24166667 0.24583333 0.25 0.25416667 0.25833333 0.2625 0.26666667 0.27083333 0.275 0.27916667 0.28333333 0.2875 0.29166667 0.29583333 0.3 0.30416667 0.30833333 0.3125 0.31666667 0.32083333 0.325 0.32916667 0.33333333 0.3375 0.34166667 0.34583333 0.35 0.35416667 0.35833333 0.3625 0.36666667 0.37083333 0.375 0.37916667 0.38333333 0.3875 0.39166667 0.39583333 0.4 0.40416667 0.40833333 0.4125 0.41666667 0.42083333 0.425 0.42916667 0.43333333 0.4375 0.44166667 0.44583333 0.45 0.45416667 0.45833333 0.4625 0.46666667 0.47083333 0.475 0.47916667 0.48333333 0.4875 0.49166667 0.49583333 0.5 0.50416667 0.50833333 0.5125 0.51666667 0.52083333 0.525 0.52916667 0.53333333 0.5375 0.54166667 0.54583333 0.55 0.55416667 0.55833333 0.5625 0.56666667 0.57083333 0.575 0.57916667 0.58333333 0.5875 0.59166667 0.59583333 0.6 0.60416667 0.60833333 0.6125 0.61666667 0.62083333 0.625 0.62916667 0.63333333 0.6375 0.64166667 0.64583333 0.65 0.65416667 0.65833333 0.6625 0.66666667 0.67083333 0.675 0.67916667 0.68333333 0.6875 0.69166667 0.69583333 0.7 0.70416667 0.70833333 0.7125 0.71666667 0.72083333 0.725 0.72916667 0.73333333 0.7375 0.74166667 0.74583333 0.75 0.75416667 0.75833333 0.7625 0.76666667 0.77083333 0.775 0.77916667 0.78333333 0.7875 0.79166667 0.79583333 0.8 0.80416667 0.80833333 0.8125 0.81666667 0.82083333 0.825 0.82916667 0.83333333 0.8375 0.84166667 0.84583333 0.85 0.85416667 0.85833333 0.8625 0.86666667 0.87083333 0.875 0.87916667 0.88333333 0.8875 0.89166667 0.89583333 0.9 0.90416667 0.90833333 0.9125 0.91666667 0.92083333 0.925 0.92916667 0.93333333 0.9375 0.94166667 0.94583333 0.95 0.95416667 0.95833333 0.9625 0.96666667 0.97083333 0.975 0.97916667 0.98333333 0.9875 0.99166667 0.99583333 1 1 1 1 1 1
  arc A23 (-18.6136, -12.2898) -> (-17.8246, -12.863) centre (0, 12.5) ccw
  spline S23 degree 5 poles (-17.8246, -12.863) (-17.8224, -12.8615) (-17.8179, -12.8584) (-17.8112, -12.8539) (-17.8023, -12.8477) (-17.7913, -12.8401) (-17.7802, -12.8325) (-17.7692, -12.8248) (-17.7583, -12.8172) (-17.7473, -12.8096) (-17.7364, -12.8019) (-17.7256, -12.7943) (-17.7147, -12.7867) (-17.7039, -12.7791) (-17.6932, -12.7715) (-17.6825, -12.7639) (-17.6718, -12.7563) (-17.6611, -12.7487) (-17.6505, -12.7411) (-17.6399, -12.7335) (-17.6294, -12.7259) (-17.6189, -12.7184) (-17.6084, -12.7108) (-17.598, -12.7032) (-17.5876, -12.6957) (-17.5772, -12.6881) (-17.5669, -12.6806) (-17.5566, -12.6731) (-17.5464, -12.6655) (-17.5361, -12.658) (-17.526, -12.6505) (-17.5158, -12.643) (-17.5057, -12.6355) (-17.4956, -12.628) (-17.4856, -12.6205) (-17.4756, -12.613) (-17.4657, -12.6055) (-17.4557, -12.5981) (-17.4458, -12.5906) (-17.436, -12.5832) (-17.4262, -12.5757) (-17.4164, -12.5683) (-17.4067, -12.5609) (-17.397, -12.5534) (-17.3873, -12.546) (-17.3777, -12.5386) (-17.3681, -12.5312) (-17.3585, -12.5238) (-17.349, -12.5165) (-17.3395, -12.5091) (-17.3301, -12.5017) (-17.3207, -12.4944) (-17.3113, -12.4871) (-17.302, -12.4797) (-17.2927, -12.4724) (-17.2835, -12.4651) (-17.2743, -12.4578) (-17.2651, -12.4505) (-17.2559, -12.4432) (-17.2469, -12.436) (-17.2378, -12.4287) (-17.2288, -12.4215) (-17.2198, -12.4142) (-17.2108, -12.407) (-17.2019, -12.3998) (-17.1931, -12.3926) (-17.1842, -12.3854) (-17.1754, -12.3782) (-17.1667, -12.3711) (-17.158, -12.3639) (-17.1493, -12.3568) (-17.1407, -12.3496) (-17.1321, -12.3425) (-17.1235, -12.3354) (-17.115, -12.3283) (-17.1065, -12.3212) (-17.0981, -12.3142) (-17.0897, -12.3071) (-17.0813, -12.3001) (-17.073, -12.2931) (-17.0647, -12.2861) (-17.0565, -12.2791) (-17.0483, -12.2721) (-17.0401, -12.2651) (-17.032, -12.2582) (-17.0239, -12.2512) (-17.0159, -12.2443) (-17.0079, -12.2374) (-16.9999, -12.2305) (-16.992, -12.2236) (-16.9841, -12.2168) (-16.9763, -12.2099) (-16.9685, -12.2031) (-16.9607, -12.1963) (-16.953, -12.1895) (-16.9453, -12.1827) (-16.9377, -12.1759) (-16.9301, -12.1692) (-16.9225, -12.1625) (-16.915, -12.1558) (-16.9075, -12.1491) (-16.9001, -12.1424) (-16.8927, -12.1357) (-16.8854, -12.1291) (-16.8781, -12.1225) (-16.8708, -12.1159) (-16.8636, -12.1093) (-16.8564, -12.1027) (-16.8492, -12.0962) (-16.8421, -12.0897) (-16.8351, -12.0831) (-16.8281, -12.0767) (-16.8211, -12.0702) (-16.8142, -12.0638) (-16.8073, -12.0573) (-16.8004, -12.0509) (-16.7936, -12.0446) (-16.7869, -12.0382) (-16.7801, -12.0319) (-16.7735, -12.0255) (-16.7668, -12.0192) (-16.7602, -12.013) (-16.7537, -12.0067) (-16.7472, -12.0005) (-16.7407, -11.9943) (-16.7343, -11.9881) (-16.7279, -11.982) (-16.7216, -11.9758) (-16.7153, -11.9697) (-16.7091, -11.9636) (-16.7029, -11.9576) (-16.6967, -11.9515) (-16.6906, -11.9455) (-16.6845, -11.9395) (-16.6785, -11.9336) (-16.6725, -11.9277) (-16.6666, -11.9218) (-16.6607, -11.9159) (-16.6549, -11.91) (-16.6491, -11.9042) (-16.6433, -11.8984) (-16.6376, -11.8926) (-16.6319, -11.8869) (-16.6263, -11.8812) (-16.6207, -11.8755) (-16.6152, -11.8698) (-16.6097, -11.8642) (-16.6043, -11.8586) (-16.5989, -11.853) (-16.5935, -11.8475) (-16.5882, -11.842) (-16.583, -11.8365) (-16.5778, -11.8311) (-16.5726, -11.8257) (-16.5675, -11.8203) (-16.5624, -11.8149) (-16.5574, -11.8096) (-16.5524, -11.8043) (-16.5475, -11.7991) (-16.5426, -11.7939) (-16.5378, -11.7887) (-16.533, -11.7835) (-16.5282, -11.7784) (-16.5236, -11.7733) (-16.5189, -11.7683) (-16.5143, -11.7633) (-16.5098, -11.7583) (-16.5053, -11.7534) (-16.5008, -11.7485) (-16.4964, -11.7436) (-16.492, -11.7388) (-16.4877, -11.734) (-16.4835, -11.7293) (-16.4793, -11.7246) (-16.4751, -11.7199) (-16.471, -11.7153) (-16.4669, -11.7107) (-16.4629, -11.7062) (-16.459, -11.7017) (-16.455, -11.6972) (-16.4512, -11.6928) (-16.4474, -11.6884) (-16.4436, -11.6841) (-16.4399, -11.6798) (-16.4362, -11.6755) (-16.4326, -11.6713) (-16.4291, -11.6672) (-16.4256, -11.6631) (-16.4221, -11.659) (-16.4187, -11.655) (-16.4153, -11.651) (-16.412, -11.6471) (-16.4088, -11.6432) (-16.4056, -11.6394) (-16.4024, -11.6356) (-16.3994, -11.6319) (-16.3963, -11.6283) (-16.3933, -11.6246) (-16.3904, -11.6211) (-16.3875, -11.6176) (-16.3847, -11.6141) (-16.3819, -11.6107) (-16.3792, -11.6073) (-16.3766, -11.604) (-16.374, -11.6008) (-16.3714, -11.5976) (-16.3689, -11.5945) (-16.3665, -11.5914) (-16.3641, -11.5884) (-16.3618, -11.5855) (-16.3595, -11.5826) (-16.3573, -11.5798) (-16.3551, -11.577) (-16.353, -11.5743) (-16.351, -11.5717) (-16.349, -11.5691) (-16.3471, -11.5666) (-16.3452, -11.5641) (-16.3434, -11.5618) (-16.3416, -11.5595) (-16.3399, -11.5572) (-16.3383, -11.5551) (-16.3367, -11.553) (-16.3352, -11.551) (-16.3338, -11.549) (-16.3324, -11.5471) (-16.331, -11.5453) (-16.3298, -11.5436) (-16.3286, -11.542) (-16.3274, -11.5404) (-16.3263, -11.5389) (-16.3253, -11.5375) (-16.3244, -11.5362) (-16.3235, -11.535) (-16.3227, -11.5338) (-16.3219, -11.5327) (-16.3212, -11.5317) (-16.3206, -11.5309) (-16.32, -11.5301) (-16.3195, -11.5294) (-16.3191, -11.5287) (-16.3188, -11.5283) (-16.3186, -11.5281) (-16.3185, -11.5279) (-16.3184, -11.5278) knots -1 -1 -1 -1 -1 -1 -0.99583333 -0.99166667 -0.9875 -0.98333333 -0.97916667 -0.975 -0.97083333 -0.96666667 -0.9625 -0.95833333 -0.95416667 -0.95 -0.94583333 -0.94166667 -0.9375 -0.93333333 -0.92916667 -0.925 -0.92083333 -0.91666667 -0.9125 -0.90833333 -0.90416667 -0.9 -0.89583333 -0.89166667 -0.8875 -0.88333333 -0.87916667 -0.875 -0.87083333 -0.86666667 -0.8625 -0.85833333 -0.85416667 -0.85 -0.84583333 -0.84166667 -0.8375 -0.83333333 -0.82916667 -0.825 -0.82083333 -0.81666667 -0.8125 -0.80833333 -0.80416667 -0.8 -0.79583333 -0.79166667 -0.7875 -0.78333333 -0.77916667 -0.775 -0.77083333 -0.76666667 -0.7625 -0.75833333 -0.75416667 -0.75 -0.74583333 -0.74166667 -0.7375 -0.73333333 -0.72916667 -0.725 -0.72083333 -0.71666667 -0.7125 -0.70833333 -0.70416667 -0.7 -0.69583333 -0.69166667 -0.6875 -0.68333333 -0.67916667 -0.675 -0.67083333 -0.66666667 -0.6625 -0.65833333 -0.65416667 -0.65 -0.64583333 -0.64166667 -0.6375 -0.63333333 -0.62916667 -0.625 -0.62083333 -0.61666667 -0.6125 -0.60833333 -0.60416667 -0.6 -0.59583333 -0.59166667 -0.5875 -0.58333333 -0.57916667 -0.575 -0.57083333 -0.56666667 -0.5625 -0.55833333 -0.55416667 -0.55 -0.54583333 -0.54166667 -0.5375 -0.53333333 -0.52916667 -0.525 -0.52083333 -0.51666667 -0.5125 -0.50833333 -0.50416667 -0.5 -0.49583333 -0.49166667 -0.4875 -0.48333333 -0.47916667 -0.475 -0.47083333 -0.46666667 -0.4625 -0.45833333 -0.45416667 -0.45 -0.44583333 -0.44166667 -0.4375 -0.43333333 -0.42916667 -0.425 -0.42083333 -0.41666667 -0.4125 -0.40833333 -0.40416667 -0.4 -0.39583333 -0.39166667 -0.3875 -0.38333333 -0.37916667 -0.375 -0.37083333 -0.36666667 -0.3625 -0.35833333 -0.35416667 -0.35 -0.34583333 -0.34166667 -0.3375 -0.33333333 -0.32916667 -0.325 -0.32083333 -0.31666667 -0.3125 -0.30833333 -0.30416667 -0.3 -0.29583333 -0.29166667 -0.2875 -0.28333333 -0.27916667 -0.275 -0.27083333 -0.26666667 -0.2625 -0.25833333 -0.25416667 -0.25 -0.24583333 -0.24166667 -0.2375 -0.23333333 -0.22916667 -0.225 -0.22083333 -0.21666667 -0.2125 -0.20833333 -0.20416667 -0.2 -0.19583333 -0.19166667 -0.1875 -0.18333333 -0.17916667 -0.175 -0.17083333 -0.16666667 -0.1625 -0.15833333 -0.15416667 -0.15 -0.14583333 -0.14166667 -0.1375 -0.13333333 -0.12916667 -0.125 -0.12083333 -0.11666667 -0.1125 -0.10833333 -0.10416667 -0.1 -0.09583333 -0.09166667 -0.0875 -0.08333333 -0.07916667 -0.075 -0.07083333 -0.06666667 -0.0625 -0.05833333 -0.05416667 -0.05 -0.04583333 -0.04166667 -0.0375 -0.03333333 -0.02916667 -0.025 -0.02083333 -0.01666667 -0.0125 -0.00833333 -0.00416667 0 0 0 0 0 0
  line L55 (-16.3184, -11.5278) -> (-16.318, -11.5271)
  line L56 (-16.318, -11.5271) -> (-16.1526, -11.2836)
  arc A24 (-16.1526, -11.2836) -> (-15.1575, -11.9297) centre (0, 12.5) ccw
  line L57 (-15.1575, -11.9297) -> (-15.3128, -12.1799)
  line L58 (-15.3128, -12.1799) -> (-15.3132, -12.1806)